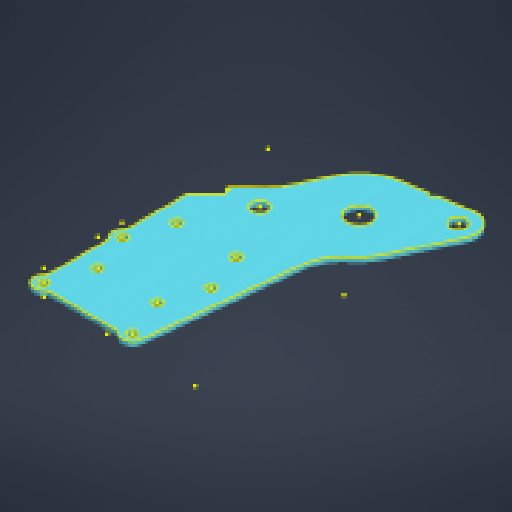
# Autodesk Inventor part: femur_support_steel
Saved by Autodesk Inventor 2026 (Build 300175000, 175)
## iProperties
Created: 2026-04-24
Part Number: femur_support_steel
Material: Сталь
Document SubType Name: Modeling
Designer: user
Density: 7.85 g/cm^3
Appearance: Серо-синий
Mass: 237.917 g
Surface Area: 222.677 cm^2
Volume: 30.3078 cm^3
Author: user
Autodesk Inventor part; units mm, degrees
ref_plane "YZ Plane" through (0, 0, 0) normal (1, 0, 0) x (0, 1, 0)
ref_plane "XZ Plane" through (0, 0, 0) normal (0, 1, 0) x (-1, 0, 0)
ref_plane "XY Plane" through (0, 0, 0) normal (0, 0, 1) x (1, 0, 0)
sketch "Эскиз1" plane through (0, 0, 0) normal (0, 1, 0) x (-1, 0, 0)
  arc A0 (40.3387, -155.9498) -> (43.3926, -135.6785) centre (41.8656, -145.8142) ccw
  line L0 (111.6413, -108.8142) -> (38.7953, -108.8142) construction
  line L1 (76.8656, 21.9817) -> (76.8656, -112.0617)
  circle A1 centre (48.8156, -8.8142) radius 3.05
  circle A2 centre (57.9156, -33.8142) radius 3.05
  circle A3 centre (48.8156, -58.8142) radius 3.05
  circle A4 centre (57.9156, -83.8142) radius 3.05
  circle A5 centre (95.8156, -83.8142) radius 3.05
  circle A6 centre (104.9156, -58.8142) radius 3.05
  circle A7 centre (95.8156, -33.8142) radius 3.05
  circle A8 centre (104.9156, -8.8142) radius 3.05
  arc A9 (53.0155, -4.3903) -> (42.8334, -7.6214) centre (48.8156, -8.8142) ccw
  arc A10 (109.3395, -13.0141) -> (100.7157, -4.3903) centre (104.9156, -8.8142) ccw
  arc A11 (109.3395, -63.0141) -> (109.3395, -54.6142) centre (104.9156, -58.8142) ccw
  line L2 (107.9656, -102.3962) -> (107.9656, -66.4566)
  line L3 (107.9656, -51.1717) -> (107.9656, -16.4566)
  line L4 (97.2731, -5.7642) -> (56.4581, -5.7642)
  line L5 (28.3919, -80.0515) -> (42.8334, -7.6214)
  circle A12 centre (41.8656, -145.8142) radius 18 construction
  line L6 (101.8656, -108.8142) -> (101.8656, -72.3334) construction
  line L7 (101.8656, -108.8142) -> (33.562, -180.6784) construction
  line L8 (51.8656, -108.8142) -> (51.8656, -72.3334) construction
  line L9 (96.2539, -114.7184) -> (107.9656, -102.3962)
  line L10 (96.2539, -114.7184) -> (99.1818, -117.5012)
  arc A13 (98.953, -120.5879) -> (99.1818, -117.5012) centre (97.804, -118.9509) ccw
  circle A14 centre (41.8656, -145.8142) radius 45.2548 construction
  circle A15 centre (14.9897, -109.4042) radius 5.05
  circle A16 centre (5.4556, -172.69) radius 5.05
  arc A17 (-5.4216, -171.0513) -> (3.8169, -183.5673) centre (5.4556, -172.69) ccw
  line L11 (98.953, -120.5879) -> (87.305, -132.8431)
  arc A18 (109.3395, -63.0141) -> (107.9656, -66.4566) centre (112.9656, -66.4566) ccw
  arc A19 (107.9656, -51.1717) -> (109.3395, -54.6142) centre (112.9656, -51.1717) ccw
  arc A20 (109.3395, -13.0141) -> (107.9656, -16.4566) centre (112.9656, -16.4566) ccw
  arc A21 (97.2731, -5.7642) -> (100.7157, -4.3903) centre (97.2731, -0.7642) ccw
  arc A22 (53.0155, -4.3903) -> (56.4581, -5.7642) centre (56.4581, -0.7642) ccw
  circle A23 centre (68.7415, -182.2241) radius 5.05
  circle A24 centre (78.2756, -118.9383) radius 5.05
  arc A25 (67.1028, -193.1014) -> (79.6187, -183.8628) centre (68.7415, -182.2241) ccw
  arc A26 (11.5934, -98.9416) -> (4.1125, -107.7655) centre (14.9897, -109.4042) ccw
  line L12 (78.2756, -118.9383) -> (78.2756, -108.8142) construction
  line L13 (78.2756, -118.9383) -> (85.6139, -125.913) construction
  line L14 (67.1028, -193.1014) -> (3.8169, -183.5673)
  line L15 (79.6187, -183.8628) -> (87.305, -132.8431)
  arc A27 (82.6506, -129.0308) -> (83.6843, -128.5167) centre (78.2756, -118.9383) ccw
  arc A28 (11.5934, -98.9416) -> (28.3919, -80.0515) centre (3.8745, -75.1631) ccw
  line L16 (43.3926, -135.6785) -> (0.8724, -129.2728)
  line L17 (40.3387, -155.9498) -> (-2.1815, -149.544)
  line L18 (4.1125, -107.7655) -> (0.8724, -129.2728)
  line L19 (-2.1815, -149.544) -> (-5.4216, -171.0513)
  line L20 (33.562, -180.6784) -> (35.8815, -182.8829)
  line L21 (35.8815, -182.8829) -> (31.2963, -187.7071)
  line L22 (33.562, -180.6784) -> (27.4345, -187.1253)
  point P0 (0, 0)
  point P1 (107.9656, -64.0969)
  point P2 (107.9656, -53.5314)
  point P3 (107.9656, -14.0969)
  point P4 (99.6329, -5.7642)
  point P5 (54.0984, -5.7642)
  point P6 (100.603, -118.8519)
  point P7 (21.7907, -113.1589)
  point P8 (80.5833, -139.9152)
  point P9 (85.6933, -134.5388)
  dimension "d4" = 37.9
  dimension "d5" = 56.1
  dimension "d6" = 6.1
  dimension "d7" = 50
  dimension "d8" = 50
  dimension "d9" = 25
  dimension "d10" = 50
  dimension "d11" = 37.9
  dimension "d12" = 56.1
  dimension "d15" = 35
  dimension "d16" = 37
  dimension "d17" = 20.5
  dimension "d20" = 12.2
  dimension "d21" = 12.2
  dimension "d24" = 3.05
  dimension "d26" = 36
  dimension "d29" = 50
  dimension "d33" = 10.1
  dimension "d36" = 360
  dimension "d38" = 64
  dimension "d44" = 22
  dimension "d45" = 6
  dimension "d49" = 17
  dimension "d52" = 5
  dimension "d54" = 25
  dimension "d55" = 3.2
  dimension "d56" = 91
  constraints: 46 end point, 38 point on circle, 29 centre point, 25 tangent, 19 point on line, 14 equal radius, 11 perpendicular, 9 coincident, 4 horizontal alignment, 4 vertical alignment, 2 parallel, 2 symmetric about line, 2 vertical, 1 equal length, 10 other
  measures "d4" distance of A5.centre A4.centre
  measures "d5" distance of A8.centre A1.centre
  measures "d6" diameter of A1
  measures "d7" distance from line of A3.centre L0
  measures "d8" distance of A1.centre A3.centre
  measures "d9" distance from line of L0 A4.centre
  measures "d10" distance of A2.centre A4.centre
  measures "d11" diameter of A2.centre L1
  measures "d12" diameter of A1.centre L1
  measures "d15" distance from line of A0.centre L1
  measures "d16" distance from line of L0 A0.centre
  measures "d17" diameter of A0
  measures "d20" diameter of A10
  measures "d21" diameter of A11
  measures "d24" distance from line of L4 A8.centre
  measures "d26" diameter of A12
  measures "d29" diameter of L6 L1
  measures "d33" diameter of A15
  measures "d38" distance of A16.centre A15.centre
  measures "d44" diameter of A17
  measures "d45" distance between parallel lines of L11 L7
  measures "d49" distance from line of L10 L2.start
  measures "d52" radius of A18
  measures "d54" radius of A28
  measures "d55" distance of L7.end L20.end
  measures "d56" distance between parallel lines of L20 L10
extrude "Выдавливание1" add sketch "Эскиз1" along normal blind 3 contours A0 L16 L18 A26 A28 L5 A9 A22 L4 A21 A10 A20 L3 A19 A11 A18 L2 L9 L10 A13 L11 L15 A25 L14 L21 L20 L22 A17 L19 L17
sketch "Эскиз2" plane through (0, 3, 0) normal (0, 1, 0) x (1, 0, 0)
  line L0 (-107.9656, 102.3962) -> (-107.9656, 66.4566) projected
  arc A0 (-109.3395, 63.0141) -> (-109.3395, 54.6142) centre (-104.9156, 58.8142) ccw projected
  line L1 (-107.9656, 51.1717) -> (-107.9656, 16.4566) projected
  arc A1 (-109.3395, 13.0141) -> (-100.7157, 4.3903) centre (-104.9156, 8.8142) ccw projected
  line L2 (-97.2731, 5.7642) -> (-56.4581, 5.7642) projected
  arc A2 (-53.0155, 4.3903) -> (-42.8334, 7.6214) centre (-48.8156, 8.8142) ccw projected
  line L3 (-42.8334, 7.6214) -> (-28.3919, 80.0515) projected
  arc A3 (5.4216, 171.0513) -> (-3.8169, 183.5673) centre (-5.4556, 172.69) ccw projected
  line L4 (-87.305, 132.8431) -> (-98.953, 120.5879) projected
  arc A4 (-98.953, 120.5879) -> (-99.1818, 117.5012) centre (-97.804, 118.9509) ccw projected
  line L5 (-99.1818, 117.5012) -> (-96.2539, 114.7184) projected
  line L6 (-96.2539, 114.7184) -> (-107.9656, 102.3962) projected
  circle A5 centre (-95.8156, 33.8142) radius 3.05 projected
  circle A6 centre (-95.8156, 83.8142) radius 3.05 projected
  circle A7 centre (-57.9156, 83.8142) radius 3.05 projected
  circle A8 centre (-48.8156, 58.8142) radius 3.05 projected
  circle A9 centre (-57.9156, 33.8142) radius 3.05 projected
  arc A10 (-40.3387, 155.9498) -> (-43.3926, 135.6785) centre (-41.8656, 145.8142) ccw projected
  circle A11 centre (-5.4556, 172.69) radius 5.05 projected
  circle A12 centre (-14.9897, 109.4042) radius 5.05 projected
  circle A13 centre (-104.9156, 8.8142) radius 3.05 projected
  circle A14 centre (-104.9156, 58.8142) radius 3.05 projected
  circle A15 centre (-48.8156, 8.8142) radius 3.05 projected
  arc A16 (-109.3395, 63.0141) -> (-107.9656, 66.4566) centre (-112.9656, 66.4566) ccw projected
  arc A17 (-107.9656, 51.1717) -> (-109.3395, 54.6142) centre (-112.9656, 51.1717) ccw projected
  arc A18 (-109.3395, 13.0141) -> (-107.9656, 16.4566) centre (-112.9656, 16.4566) ccw projected
  arc A19 (-97.2731, 5.7642) -> (-100.7157, 4.3903) centre (-97.2731, 0.7642) ccw projected
  arc A20 (-53.0155, 4.3903) -> (-56.4581, 5.7642) centre (-56.4581, 0.7642) ccw projected
  arc A21 (-11.5934, 98.9416) -> (-28.3919, 80.0515) centre (-3.8745, 75.1631) ccw projected
  arc A22 (-11.5934, 98.9416) -> (-4.1125, 107.7655) centre (-14.9897, 109.4042) ccw projected
  line L7 (-4.1125, 107.7655) -> (-0.8724, 129.2728) projected
  line L8 (-0.8724, 129.2728) -> (-43.3926, 135.6785) projected
  line L9 (-40.3387, 155.9498) -> (2.1815, 149.544) projected
  line L10 (2.1815, 149.544) -> (5.4216, 171.0513) projected
  line L11 (-3.8169, 183.5673) -> (-27.4345, 187.1253) projected
  arc A23 (-67.1028, 193.1014) -> (-79.6187, 183.8628) centre (-68.7415, 182.2241) ccw projected
  line L12 (-79.6187, 183.8628) -> (-87.305, 132.8431) projected
  line L13 (-27.4345, 187.1253) -> (-33.562, 180.6784) projected
  line L14 (-33.562, 180.6784) -> (-35.8815, 182.8829) projected
  line L15 (-35.8815, 182.8829) -> (-31.2963, 187.7071) projected
  line L16 (-31.2963, 187.7071) -> (-67.1028, 193.1014) projected
  point P0 (0, 0)
equation "\"d4\" = -d_main_screw_holes + hight_profile_femur - 2 * thickness_profile_femur"
equation "\"d5\" = hight_profile_femur + d_main_screw_holes"
equation "\"d6\" = d_main_screw_holes"
equation "\"d11\" = -d_main_screw_holes + hight_profile_femur - 2 * thickness_profile_femur"
equation "\"d12\" = hight_profile_femur + d_main_screw_holes"
equation "\"d15\" = width_shaft_shift"
equation "\"d20\" = 2 * d_main_screw_holes"
equation "\"d21\" = 2 * d_main_screw_holes"
equation "\"d24\" = 0.5 * d_main_screw_holes"
equation "\"d29\" = width_profile_femur"
equation "\"d2\" = thickness_steel"
equation "\"tolerance_plazma\" = 0.1"
equation "\"thickness_steel\" = 3"
equation "\"d_main_screw_holes\" = 6.1"
equation "\"thickness_profile_tibea\" = 3"
equation "\"hight_shaft_shift\" = 37"
equation "\"thickness_profile_femur\" = 3"
equation "\"width_profile_femur\" = 50"
equation "\"width_shaft_shift\" = 35"
equation "\"hight_profile_femur\" = 50"
equation "\"width_flattened_surface\" = 12"
